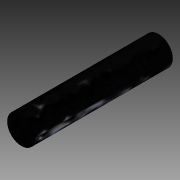
# Autodesk Inventor part: Igus Rod
Saved by Autodesk Inventor 2014 (Build 180170000, 170)
## iProperties
Created: 2015-02-07
Part Number: Igus Rod
Material: Generic
Document SubType Name: Modeling
Designer: Spooner
Density: 1 g/cm^3
Appearance: Black
Author: Spooner
Autodesk Inventor part; units mm, degrees
ref_plane "YZ Plane" through (0, 0, 0) normal (1, 0, 0) x (0, 1, 0)
ref_plane "XZ Plane" through (0, 0, 0) normal (0, 1, 0) x (-1, 0, 0)
ref_plane "XY Plane" through (0, 0, 0) normal (0, 0, 1) x (1, 0, 0)
sketch "Sketch1" plane through (0, 0, 0) normal (0, 0, 1) x (1, 0, 0)
  circle A0 centre (0, 0) radius 7.874
  dimension "d0" = 15.748
  constraints: 1 centre point, 1 coincident
  measures "d0" diameter of A0
extrude "Extrusion1" add sketch "Sketch1" along normal blind 76.2
body "Solid1"
